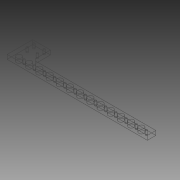
# Autodesk Inventor part: Set Square
Saved by Autodesk Inventor 2012 (Build 160160000, 160)
## iProperties
Created: 2013-02-20
Part Number: Set Square
Material: Default
Document SubType Name: Modeling
Designer: mce
Density: 1 g/cm^3
Mass: 82.3969 g
Surface Area: 247.653 cm^2
Volume: 82.3969 cm^3
Author: mce
Autodesk Inventor part; units mm, degrees
ref_plane "YZ Plane" through (0, 0, 0) normal (1, 0, 0) x (0, 1, 0)
ref_plane "XZ Plane" through (0, 0, 0) normal (0, 1, 0) x (-1, 0, 0)
ref_plane "XY Plane" through (0, 0, 0) normal (0, 0, 1) x (1, 0, 0)
sketch "Sketch1" plane through (0, 0, 0) normal (0, 0, 1) x (1, 0, 0)
  line L0 (0, 0) -> (18.2608, 0)
  line L1 (42, 25) -> (42, 60)
  line L2 (42, 60) -> (0, 60)
  line L3 (0, 60) -> (0, 0)
  line L4 (47, 20) -> (330, 20)
  line L5 (330, 20) -> (330, 0)
  line L6 (330, 0) -> (18.2608, 0)
  circle A0 centre (9, 54) radius 2.05
  circle A1 centre (33, 54) radius 2.05
  circle A2 centre (33, 38) radius 2.05
  circle A3 centre (9, 38) radius 2.05
  line L7 (42, 25) -> (47, 20)
  point P0 (42, 20)
  dimension "d0" = 330
  dimension "d1" = 60
  dimension "d2" = 42
  dimension "d3" = 40
  dimension "d4" = 4.1
  dimension "d5" = 24
  dimension "d6" = 16
  dimension "d7" = 6
  dimension "d8" = 9
  dimension "d9" = 5
  dimension "d10" = 5
  constraints: 16 end point, 4 centre point, 3 equal radius, 2 horizontal alignment, 2 point on line, 2 vertical alignment, 1 collinear, 1 horizontal, 1 vertical
  measures "d0" distance between parallel lines of L5 L3
  measures "d1" distance between parallel lines of L2 L0
  measures "d2" distance between parallel lines of L3 L1
  measures "d3" distance between parallel lines of L2 L4
  measures "d4" diameter of A0
  measures "d5" distance of A1.centre A0.centre
  measures "d6" distance of A0.centre A3.centre
  measures "d7" distance from line of L2 A0.centre
  measures "d8" distance from line of L3 A0.centre
  measures "d9" distance of L1.start point (42, 20)
  measures "d10" distance of L4.start point (42, 20)
extrude "Extrusion1" add sketch "Sketch1" along normal blind 10
sketch "Sketch2" plane through (0, 0, 10) normal (0, 0, 1) x (1, 0, 0)
  line L0 (330, 20) -> (330, 0) projected
  line L1 (47, 20) -> (330, 20) projected
  circle A0 centre (318, 10) radius 2
  circle A1 centre (306, 10) radius 6
  line L2 (336.598, 10) -> (-63.669, 10) construction
  circle A2 centre (294, 10) radius 2
  circle A3 centre (282, 10) radius 6
  line L3 (312.598, 10) -> (-87.669, 10) construction
  circle A4 centre (270, 10) radius 2
  circle A5 centre (258, 10) radius 6
  line L4 (288.598, 10) -> (-111.669, 10) construction
  circle A6 centre (246, 10) radius 2
  circle A7 centre (234, 10) radius 6
  line L5 (264.598, 10) -> (-135.669, 10) construction
  circle A8 centre (222, 10) radius 2
  circle A9 centre (210, 10) radius 6
  line L6 (240.598, 10) -> (-159.669, 10) construction
  circle A10 centre (198, 10) radius 2
  circle A11 centre (186, 10) radius 6
  line L7 (216.598, 10) -> (-183.669, 10) construction
  circle A12 centre (174, 10) radius 2
  circle A13 centre (162, 10) radius 6
  line L8 (192.598, 10) -> (-207.669, 10) construction
  circle A14 centre (150, 10) radius 2
  circle A15 centre (138, 10) radius 6
  line L9 (168.598, 10) -> (-231.669, 10) construction
  circle A16 centre (126, 10) radius 2
  circle A17 centre (114, 10) radius 6
  line L10 (144.598, 10) -> (-255.669, 10) construction
  circle A18 centre (102, 10) radius 2
  circle A19 centre (90, 10) radius 6
  line L11 (120.598, 10) -> (-279.669, 10) construction
  circle A20 centre (78, 10) radius 2
  circle A21 centre (66, 10) radius 6
  line L12 (96.598, 10) -> (-303.669, 10) construction
  circle A22 centre (54, 10) radius 2
  circle A23 centre (42, 10) radius 6
  line L13 (72.598, 10) -> (-327.669, 10) construction
  circle A24 centre (30, 10) radius 2
  circle A25 centre (18, 10) radius 6
  line L14 (48.598, 10) -> (-351.669, 10) construction
  dimension "d13" = 10
  dimension "d14" = 12
  dimension "d15" = 4
  dimension "d16" = 12
  dimension "d17" = 12
  dimension "d20" = 24
  constraints: 26 centre point, 26 end point, 2 point on line, 1 collinear, 1 horizontal, 83 other
  measures "d13" distance between parallel lines of L2 L1
  measures "d14" distance of A1.centre A0.centre
  measures "d15" diameter of A0
  measures "d16" diameter of A1
  measures "d17" distance from line of L0 A0.centre
  measures "d20" distance of L2.start L3.start
extrude "Extrusion2" cut sketch "Sketch2" against normal through all
equation "\"d8\" = -0.5 * d5 + 0.5 * d2"
equation "\"d10\" = d9"
body "Solid1"
